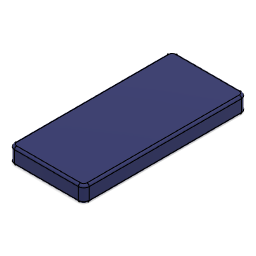
本体 v55 (Autodesk Fusion 360 archive; units mm, degrees)
design "バッテリー"
Autodesk Fusion 360 part; units mm, degrees
note: some values were not read from the file. Set by a fixed rule: which face or edge a step refers to.
sketch "スケッチ1" plane through (0, 0, 0) normal (0, 1, 0) x (1, 0, 0)
  line L0 (0, 0) -> (68.5, 0)
  line L1 (68.5, 0) -> (68.5, -149.5)
  line L2 (68.5, -149.5) -> (0, -149.5)
  line L3 (0, -149.5) -> (0, 0)
  dimension "d1" = 68.5
  dimension "d2" = 149.5
  constraint horizontal L0
  constraint vertical L1
  constraint horizontal L2
  constraint vertical L3
  constraint coincident L0.start L3.end
  measures "d1" distance of L0.start L0.end
  measures "d2" distance of L0.start L2.end
extrude "押し出し1" add sketch "スケッチ1" along normal blind 15
fillet "フィレット1" radius 5 4 edges at (68.5, 7.5, 0) (68.5, 7.5, 149.5) (0, 7.5, 149.5) (0, 7.5, 0)
fillet "フィレット2" radius 2 16 edges at (67.0355, 15, 1.4645) (34.25, 15, 0) (1.4645, 15, 1.4645) (0, 15, 74.75) (1.4645, 15, 148.0355) (34.25, 15, 149.5) (67.0355, 15, 148.0355) (68.5, 15, 74.75) (67.0355, 0, 148.0355) (34.25, 0, 149.5) (1.4645, 0, 148.0355) (0, 0, 74.75) (1.4645, 0, 1.4645) (34.25, 0, 0) (67.0355, 0, 1.4645) (68.5, 0, 74.75)
sketch "スケッチ2" plane through (0, 0, 0) normal (0, 0, -1) x (-1, 0, 0)
  line L0 (-63.5, 2) -> (-5, 2)
  line L1 (-5, 2) -> (-5, 13)
  line L2 (-5, 13) -> (-63.5, 13)
  line L3 (-63.5, 13) -> (-63.5, 2)
  line L4 (-18.8, 8.9) -> (-12.7, 8.9)
  line L5 (-11.5, 7.7) -> (-11.5, 7.3)
  line L6 (-12.7, 6.1) -> (-18.8, 6.1)
  line L7 (-20, 7.3) -> (-20, 7.7)
  line L8 (-56.5, 10.2) -> (-44.7, 10.2)
  line L9 (-44.2, 9.7) -> (-44.2, 5.3)
  line L10 (-44.7, 4.8) -> (-56.5, 4.8)
  line L11 (-57, 5.3) -> (-57, 9.7)
  line L12 (-63.5, 7.5) -> (-5, 7.5) construction
  line L13 (0, 2) -> (0, 13)
  line L14 (-68.5, 13) -> (-68.5, 2)
  arc A0 (-18.8, 8.9) -> (-20, 7.7) centre (-18.8, 7.7) ccw
  arc A1 (-20, 7.3) -> (-18.8, 6.1) centre (-18.8, 7.3) ccw
  arc A2 (-12.7, 6.1) -> (-11.5, 7.3) centre (-12.7, 7.3) ccw
  arc A3 (-11.5, 7.7) -> (-12.7, 8.9) centre (-12.7, 7.7) ccw
  arc A4 (-44.2, 9.7) -> (-44.7, 10.2) centre (-44.7, 9.7) ccw
  arc A5 (-44.7, 4.8) -> (-44.2, 5.3) centre (-44.7, 5.3) ccw
  arc A6 (-57, 5.3) -> (-56.5, 4.8) centre (-56.5, 5.3) ccw
  arc A7 (-56.5, 10.2) -> (-57, 9.7) centre (-56.5, 9.7) ccw
  point P0 (-20, 8.9)
  point P1 (-11.5, 8.9)
  point P2 (-11.5, 6.1)
  point P3 (-57, 10.2)
  point P4 (-44.2, 10.2)
  point P5 (-44.2, 4.8)
  dimension "d7" = 11.5
  dimension "d8" = 11.5
  dimension "d9" = 8.5
  dimension "d10" = 2.8
  dimension "d11" = 1.2
  dimension "d12" = 12.8
  dimension "d13" = 5.4
  dimension "d14" = 0.5
  constraint horizontal L4
  constraint vertical L5
  constraint horizontal L6
  constraint vertical L7
  constraint horizontal L8
  constraint vertical L9
  constraint horizontal L10
  constraint vertical L11
  constraint midpoint L3 L12.start
  constraint midpoint L1 L12.end
  constraint symmetric L4 L6 L12
  constraint symmetric L8 L10 L12
  constraint coincident P0 L4
  constraint coincident P0 L7
  constraint tangent L4 A0
  constraint tangent L7 A0
  constraint tangent L6 A1
  constraint tangent L7 A1
  constraint equal A0 A1
  constraint coincident P2 L5
  constraint coincident P2 L6
  constraint tangent L5 A2
  constraint tangent L6 A2
  constraint equal A0 A2
  constraint coincident P1 L4
  constraint coincident P1 L5
  constraint tangent L4 A3
  constraint tangent L5 A3
  constraint equal A0 A3
  constraint coincident P4 L8
  constraint coincident P4 L9
  constraint tangent L8 A4
  constraint tangent L9 A4
  constraint coincident P5 L9
  constraint coincident P5 L10
  constraint tangent L9 A5
  constraint tangent L10 A5
  constraint equal A4 A5
  constraint tangent L10 A6
  constraint tangent L11 A6
  constraint equal A4 A6
  constraint coincident P3 L8
  constraint coincident P3 L11
  constraint tangent L8 A7
  constraint tangent L11 A7
  constraint equal A4 A7
  measures "d7" distance of L5 L13
  measures "d8" distance of L11 L14
  measures "d9" distance of P0 P1
  measures "d10" distance of P1 P2
  measures "d11" radius of A0
  measures "d12" distance of P3 P4
  measures "d13" distance of P4 P5
  measures "d14" radius of A4
extrude "押し出し2" cut sketch "スケッチ2" against normal blind 6.5 contours L4 L5 L6 L7 A0 A1 A2 A3
extrude "押し出し3" cut sketch "スケッチ2" against normal blind 12 contours L8 L9 L10 L11 A4 A5 A6 A7

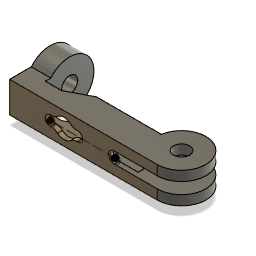
design "カメラ用マウント"
Autodesk Fusion 360 part; units mm, degrees
sketch "スケッチ1" plane through (0, 0, 0) normal (0, 1, 0) x (1, 0, 0)
  line L0 (-45.5, -7.5) -> (0, -7.5)
  circle A0 centre (0, 0) radius 2.5
  line L1 (-45.5, -7.5) -> (-45.5, 12.5)
  line L2 (-45.5, 12.5) -> (-39.5, 12.5)
  line L3 (-39.5, 12.5) -> (-39.5, -2.5)
  line L4 (-39.5, -2.5) -> (-34.5, -2.5)
  line L5 (-34.5, -2.5) -> (-27.4042, 1.1946)
  line L6 (-27.4042, 1.1946) -> (-7.4042, 1.1946)
  arc A1 (0, -7.5) -> (-7.4042, 1.1946) centre (0, 0) ccw
  line L7 (7.5, 19.5074) -> (7.5, -9) construction
  dimension "d1" = 5
  dimension "d2" = 15
  dimension "d3" = 45.5
  dimension "d4" = 20
  dimension "d5" = 6
  dimension "d6" = 5
  dimension "d7" = 8
  dimension "d8" = 20
  dimension "d9" = 5
  constraint horizontal L0
  constraint coincident A0.centre A1.centre
  constraint tangent L0 A1
  constraint perpendicular L0 L1
  constraint perpendicular L1 L2
  constraint perpendicular L2 L3
  constraint perpendicular L3 L4
  constraint parallel L4 L6
  constraint vertical L7
  constraint tangent A1 L7
  measures "d1" diameter of A0
  measures "d2" diameter of A1
  measures "d3" horizontal distance of L0.start A0.centre
  measures "d4" distance of L0 L2
  measures "d5" distance of L1.end L2.end
  measures "d6" distance of L3.end L4.end
  measures "d7" distance of L4.end L5.end
  measures "d8" distance of L5.end L6.end
  measures "d9" distance of L0 L4
extrude "押し出し1" add sketch "スケッチ1" along normal blind 9.5
sketch "スケッチ2" plane through (-45.5, 0, 0) normal (-1, 0, 0) x (0, 0, 1)
  line L0 (-12.5, 0) -> (7.5, 0)
  line L1 (7.5, 0) -> (7.5, 9.5)
  line L2 (7.5, 9.5) -> (-12.5, 9.5)
  line L3 (-12.5, 9.5) -> (-12.5, 0)
  circle A0 centre (-5, 4.75) radius 7.5
  line L4 (-12.5, 4.75) -> (7.5, 4.75) construction
  dimension "d12" = 15
  constraint tangent L3 A0
  constraint midpoint L3 L4.start
  constraint midpoint L1 L4.end
  constraint coincident A0.centre L4
  measures "d12" diameter of A0
extrude "押し出し3" cut sketch "スケッチ2" against normal up to surface (6 mm away) contours L0 L3 A0 | L2 L3 A0
extrude "押し出し2" add sketch "スケッチ2" against normal up to surface (6 mm away) contours L0 A0 | L2 A0
sketch "スケッチ3" plane through (-45.5, 0, 0) normal (-1, 0, 0) x (0, 0, 1)
  arc A0 (0.8041, 9.5) -> (0.8041, 0) centre (-5, 4.75) ccw
  line L0 (0.8041, 0) -> (7.5, 0)
  line L1 (7.5, 0) -> (7.5, 9.5)
  line L2 (7.5, 9.5) -> (0.8041, 9.5)
  circle A1 centre (-5, 4.75) radius 2.5
  dimension "d17" = 5
  constraint concentric A0 A1
  measures "d17" diameter of A1
extrude "押し出し4" cut sketch "スケッチ3" against normal up to surface (6 mm away) contours A1
sketch "スケッチ4" plane through (0, 0, 7.5) normal (0, 0, 1) x (1, 0, 0)
  line L0 (-45.5, 0) -> (0, 0)
  line L1 (0, 0) -> (0, 9.5)
  line L2 (0, 9.5) -> (-45.5, 9.5)
  line L3 (-45.5, 9.5) -> (-45.5, 0)
  line L4 (7.5, 6.5) -> (7.5, 3)
  line L5 (7.5, 3) -> (-16, 3)
  line L6 (-16, 3) -> (-13.25, 3)
  arc A0 (-13.25, 6.5) -> (-13.25, 3) centre (-13.25, 4.75) ccw
  line L7 (-13.25, 6.5) -> (7.5, 6.5)
  line L8 (0, 4.75) -> (-28.1599, 4.75) construction
  line L9 (-15, 9.5) -> (-15, 0) construction
  line L10 (7.5, 9.5) -> (-7.4042, 9.5) construction
  line L11 (7.5, 9.5) -> (7.5, 0) construction
  dimension "d20" = 3.5
  dimension "d21" = 22.5
  constraint parallel L1 L4
  constraint perpendicular L4 L5
  constraint perpendicular L4 L6
  constraint tangent L6 A0
  constraint tangent A0 L7
  constraint perpendicular L4 L7
  constraint midpoint L1 L8.start
  constraint perpendicular L1 L8
  constraint coincident L2 L9.start
  constraint coincident L0 L9.end
  constraint perpendicular L0 L9
  constraint tangent A0 L9
  constraint coincident L10.start L11.start
  constraint perpendicular L10 L11
  constraint coincident L4.start L11
  measures "d20" distance of L5 L7
  measures "d21" distance of L4 L9
extrude "押し出し5" cut sketch "スケッチ4" against normal through all contours L1 L5 A0 L7 | L1 L4 L5 L7
sketch "スケッチ5" plane through (0, 0, 7.5) normal (0, 0, 1) x (1, 0, 0)
  line L0 (0, 3) -> (-13.25, 3)
  arc A0 (-13.25, 6.5) -> (-13.25, 3) centre (-13.25, 4.75) ccw
  line L1 (-13.25, 6.5) -> (0, 6.5)
  line L2 (0, 6.5) -> (0, 9.5)
  line L3 (0, 9.5) -> (-45.5, 9.5)
  line L4 (-45.5, 9.5) -> (-45.5, 0)
  line L5 (-45.5, 0) -> (0, 0)
  line L6 (0, 0) -> (0, 3)
  line L7 (-15, 4.75) -> (-45.5, 4.75) construction
  line L8 (-23, 9.5) -> (-23, 0) construction
  line L9 (-34.5, 8.5) -> (-34.5, 0) construction
  arc A1 (-32.9093, 6.2473) -> (-32.9093, 3.2527) centre (-33, 4.75) ccw
  arc A2 (-24.5907, 3.2527) -> (-24.5907, 6.2473) centre (-24.5, 4.75) ccw
  arc A3 (-30.739, 2.5041) -> (-26.761, 2.5041) centre (-28.75, 4.75) ccw
  arc A4 (-26.761, 6.9959) -> (-30.739, 6.9959) centre (-28.75, 4.75) ccw
  arc A5 (-32.9093, 6.2473) -> (-30.739, 6.9959) centre (-32.7279, 9.2418) ccw
  arc A6 (-30.739, 2.5041) -> (-32.9093, 3.2527) centre (-32.7279, 0.2582) ccw
  arc A7 (-26.761, 6.9959) -> (-24.5907, 6.2473) centre (-24.7721, 9.2418) ccw
  arc A8 (-24.5907, 3.2527) -> (-26.761, 2.5041) centre (-24.7721, 0.2582) ccw
  dimension "d23" = 3
  dimension "d24" = 6
  dimension "d25" = 3
  dimension "d26" = 8
  dimension "d27" = 11.5
  dimension "d28" = 5.75
  dimension "d29" = 3
  constraint midpoint A0 L7.start
  constraint midpoint L4 L7.end
  constraint coincident L7 A2.centre
  constraint coincident L7 A3.centre
  constraint coincident L7 A1.centre
  constraint coincident L3 L8.start
  constraint coincident L5 L8.end
  constraint perpendicular L5 L8
  constraint tangent L8 A2
  constraint coincident L5 L9.end
  constraint perpendicular L5 L9
  constraint tangent L9 A1
  constraint concentric A3 A4
  constraint tangent A1 A5
  constraint tangent A4 A5
  constraint tangent A1 A6
  constraint tangent A3 A6
  constraint equal A5 A6
  constraint tangent A2 A7
  constraint tangent A4 A7
  constraint equal A5 A7
  constraint tangent A3 A8
  constraint tangent A2 A8
  constraint equal A5 A8
  constraint symmetric L7 A7.centre A8.centre
  measures "d23" diameter of A2
  measures "d24" diameter of A3
  measures "d25" diameter of A1
  measures "d26" distance of L7.start L8
  measures "d27" distance of L8 L9
  measures "d28" distance of A3.centre L8
  measures "d29" radius of A5
extrude "押し出し6" cut sketch "スケッチ5" against normal through all contours A1 A2 A3 A4 A5 A6 A7 A8
sketch "スケッチ6" plane through (0, 0, -1.1946) normal (0, 0, -1) x (-1, 0, 0)
  arc A0 (26.761, 2.5041) -> (27.4042, 2.0688) centre (28.75, 4.75) ccw
  arc A1 (26.761, 2.5041) -> (24.5907, 3.2527) centre (24.7721, 0.2582) ccw
  arc A2 (24.5907, 6.2473) -> (24.5907, 3.2527) centre (24.5, 4.75) ccw
  arc A3 (24.5907, 6.2473) -> (26.761, 6.9959) centre (24.7721, 9.2418) ccw
  arc A4 (27.4042, 7.4312) -> (26.761, 6.9959) centre (28.75, 4.75) ccw
  line L0 (27.4042, 7.4312) -> (27.4042, 9.5)
  line L1 (27.4042, 9.5) -> (7.4042, 9.5)
  line L2 (7.4042, 9.5) -> (7.4042, 6.5)
  line L3 (7.4042, 6.5) -> (13.25, 6.5)
  arc A5 (13.25, 3) -> (13.25, 6.5) centre (13.25, 4.75) ccw
  line L4 (13.25, 3) -> (7.4042, 3)
  line L5 (7.4042, 3) -> (7.4042, 0)
  line L6 (7.4042, 0) -> (27.4042, 0)
  line L7 (27.4042, 0) -> (27.4042, 2.0688)
  line L8 (7.4042, 8) -> (39.5, 8)
  line L9 (39.5, 8) -> (39.5, 1.5)
  line L10 (39.5, 1.5) -> (7.4042, 1.5)
  line L11 (7.4042, 1.5) -> (7.4042, 8)
  line L12 (39.5, 4.75) -> (11.4443, 4.75) construction
  line L13 (39.5, 0) -> (39.5, 9.5) construction
  point P0 (39.5, 4.75)
  dimension "d31" = 1.5
  constraint horizontal L8
  constraint vertical L9
  constraint horizontal L10
  constraint vertical L11
  constraint coincident L2 L8.start
  constraint midpoint L9 P0
  constraint perpendicular L11 L12
  constraint midpoint L13 P0
  constraint coincident P0 L12.start
  measures "d31" distance of L1 L8
extrude "押し出し7" cut sketch "スケッチ6" against normal blind 7.2 contours A0 A1 A2 A3 A4 L0 L7 L8 L9 L10 | A0 A1 A2 A3 A4 L0 L2 L3 A5 L4 L5 L7 L8 L10 L11
sketch "スケッチ7" plane through (0, 0, 7.5) normal (0, 0, 1) x (1, 0, 0)
  arc A0 (-24.5907, 3.2527) -> (-26.761, 2.5041) centre (-24.7721, 0.2582) ccw
  arc A1 (-30.739, 2.5041) -> (-26.761, 2.5041) centre (-28.75, 4.75) ccw
  arc A2 (-30.739, 2.5041) -> (-32.9093, 3.2527) centre (-32.7279, 0.2582) ccw
  arc A3 (-32.9093, 6.2473) -> (-32.9093, 3.2527) centre (-33, 4.75) ccw
  arc A4 (-32.9093, 6.2473) -> (-30.739, 6.9959) centre (-32.7279, 9.2418) ccw
  arc A5 (-26.761, 6.9959) -> (-30.739, 6.9959) centre (-28.75, 4.75) ccw
  arc A6 (-26.761, 6.9959) -> (-24.5907, 6.2473) centre (-24.7721, 9.2418) ccw
  arc A7 (-24.5907, 3.2527) -> (-24.5907, 6.2473) centre (-24.5, 4.75) ccw
  line L0 (0, 3) -> (-13.25, 3)
  arc A8 (-13.25, 6.5) -> (-13.25, 3) centre (-13.25, 4.75) ccw
  line L1 (-13.25, 6.5) -> (0, 6.5)
  line L2 (0, 6.5) -> (0, 9.5)
  line L3 (0, 9.5) -> (-45.5, 9.5)
  line L4 (-45.5, 9.5) -> (-45.5, 0)
  line L5 (-45.5, 0) -> (0, 0)
  line L6 (0, 0) -> (0, 3)
  circle A9 centre (-33, 4.75) radius 1.5 construction
  circle A10 centre (-13, 4.75) radius 1.5 construction
  line L7 (-13, 4.75) -> (-33, 4.75) construction
  dimension "d34" = 3
  dimension "d35" = 3
  dimension "d36" = 20
  constraint concentric A3 A9
  constraint coincident A10.centre L7.start
  constraint coincident A3.centre A9.centre
  constraint horizontal L7
  measures "d34" diameter of A9
  measures "d35" diameter of A10
  measures "d36" distance of A3.centre A10.centre
equation "d3 = 53 mm - 7.5 mm"
equation "d28 = ( 11.5 / 2 ) * 1 mm"

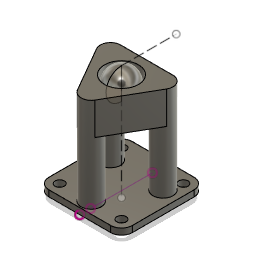
design "ボールキャスター"
Autodesk Fusion 360 part; units mm, degrees
sketch "スケッチ1" plane through (0, 0, 0) normal (0, 1, 0) x (1, 0, 0)
  line L0 (0, 0) -> (27, 0)
  line L1 (27, 0) -> (27, -27)
  line L2 (27, -27) -> (0, -27)
  line L3 (0, -27) -> (0, 0)
  dimension "d1" = 27
  dimension "d2" = 27
  constraint horizontal L0
  constraint vertical L1
  constraint horizontal L2
  constraint vertical L3
  constraint coincident L0.start L3.end
  measures "d1" distance of L0.start L2.end
  measures "d2" distance of L0.start L0.end
extrude "押し出し1" add sketch "スケッチ1" along normal blind 2
sketch "スケッチ2" plane through (0, 2, 0) normal (0, 1, 0) x (-1, 0, 0)
  line L0 (0, 27) -> (-27, 27)
  line L1 (-27, 27) -> (-27, 0)
  line L2 (-27, 0) -> (0, 0)
  line L3 (0, 0) -> (0, 27)
  circle A0 centre (-3.5, 3.5) radius 1.5
  dimension "d5" = 3
  dimension "d6" = 3.5
  dimension "d7" = 3.5
  measures "d5" diameter of A0
  measures "d6" distance of L3 A0.centre
  measures "d7" distance of L2 A0.centre
extrude "押し出し2" cut sketch "スケッチ2" against normal through all contours A0
ref_plane "作業平面1" through (13.5, 1, 15.25) normal (-1, 0, 0) x (0, 0, 1)
ref_plane "作業平面2" through (13.5, 1, 13.5) normal (0, 0, 1) x (1, 0, 0)
mirror "ミラー1" about plane through (13.5, 1, 15.25) normal (-1, 0, 0) of "押し出し2"
mirror "ミラー2" about plane through (13.5, 1, 13.5) normal (0, 0, 1) of "押し出し2", "ミラー1"
fillet "フィレット1" radius 3.5 4 edges at (27, 1, 0) (0, 1, 0) (0, 1, 27) (27, 1, 27)
sketch "スケッチ3" plane through (0, 2, 0) normal (0, 1, 0) x (-1, 0, 0)
  arc A0 (-23.5, 27) -> (-27, 23.5) centre (-23.5, 23.5) ccw
  line L0 (-27, 23.5) -> (-27, 3.5)
  arc A1 (-27, 3.5) -> (-23.5, 0) centre (-23.5, 3.5) ccw
  line L1 (-23.5, 0) -> (-3.5, 0)
  arc A2 (-3.5, 0) -> (0, 3.5) centre (-3.5, 3.5) ccw
  line L2 (0, 3.5) -> (0, 23.5)
  arc A3 (0, 23.5) -> (-3.5, 27) centre (-3.5, 23.5) ccw
  line L3 (-3.5, 27) -> (-23.5, 27)
  circle A4 centre (-23.5, 23.5) radius 1.5
  circle A5 centre (-3.5, 23.5) radius 1.5
  circle A6 centre (-23.5, 3.5) radius 1.5
  circle A7 centre (-3.5, 3.5) radius 1.5
  circle A8 centre (-22, 8.5925) radius 3.25
  circle A9 centre (-5, 8.5925) radius 3.25
  circle A10 centre (-13.5, 23.315) radius 3.25
  line L4 (-5, 8.5925) -> (-22, 8.5925) construction
  line L5 (-22, 8.5925) -> (-13.5, 23.315) construction
  line L6 (-13.5, 23.315) -> (-5, 8.5925) construction
  line L7 (0, 13.5) -> (-27, 13.5) construction
  line L8 (-13.5, 0) -> (-13.5, 27) construction
  line L9 (-5, 8.5925) -> (-17.75, 15.9537) construction
  line L10 (-22, 8.5925) -> (-9.25, 15.9537) construction
  point P0 (-13.5, 13.5)
  dimension "d12" = 6.5
  dimension "d13" = 6.5
  dimension "d14" = 6.5
  dimension "d15" = 17
  constraint coincident A9.centre L4.start
  constraint coincident A8.centre L4.end
  constraint coincident A10.centre L5.end
  constraint equal L5 L6
  constraint equal L4 L6
  constraint midpoint L2 L7.start
  constraint midpoint L0 L7.end
  constraint midpoint L1 L8.start
  constraint midpoint L3 L8.end
  constraint parallel L4 L7
  constraint coincident A10.centre L8
  constraint midpoint L5 L9.end
  constraint midpoint L6 L10.end
  constraint coincident L9 P0
  constraint coincident L10 P0
  constraint midpoint L7 P0
  measures "d12" diameter of A8
  measures "d13" diameter of A9
  measures "d14" diameter of A10
  measures "d15" distance of A8.centre A9.centre
extrude "押し出し3" add sketch "スケッチ3" along normal blind 24 contours A8 | A9 | A10
sketch "スケッチ4" plane through (0, 26, 0) normal (0, 1, 0) x (-1, 0, 0)
  circle A0 centre (-5, 8.5925) radius 3.25
  arc A1 (-5, 5.3425) -> (-2.1854, 10.2175) centre (-5, 8.5925) ccw
  line L0 (-2.1854, 10.2175) -> (-10.6854, 24.9399)
  circle A2 centre (-13.5, 23.315) radius 3.25
  arc A3 (-10.6854, 24.9399) -> (-16.3146, 24.94) centre (-13.5, 23.315) ccw
  line L1 (-5, 5.3425) -> (-22, 5.3425)
  circle A4 centre (-22, 8.5925) radius 3.25
  arc A5 (-24.8146, 10.2175) -> (-22, 5.3425) centre (-22, 8.5925) ccw
  line L2 (-24.8146, 10.2175) -> (-16.3146, 24.94)
  constraint coincident A0 A1.start
  constraint coincident A0.centre A1.centre
  constraint tangent A0 L0
  constraint tangent L0 A2
  constraint coincident A2.centre A3.centre
  constraint coincident A2 A3.end
  constraint tangent L1 A4
  constraint coincident A4 L1.end
  constraint coincident A4.centre A5.centre
  constraint tangent A4 L2
  constraint tangent A2 L2
  constraint tangent A0 L1
extrude "押し出し4" add sketch "スケッチ4" against normal blind 4
sketch "スケッチ5" plane through (13.5, 1, 15.25) normal (-1, 0, 0) x (0, 0, -1)
  line L0 (1.75, -35) -> (1.75, 1) construction
  line L1 (-11.75, -1) -> (-11.75, 1)
  line L2 (-5, -34) -> (12, -34) construction
  line L3 (11.75, 1) -> (-8.25, 1) construction
  line L4 (1.75, -34) -> (1.75, -24)
  arc A0 (1.75, -24) -> (1.75, -34) centre (1.75, -29) ccw
  dimension "d20" = 13.5
  dimension "d21" = 35
  dimension "d22" = 10
  constraint vertical L0
  constraint perpendicular L0 L2
  constraint coincident L0 L4.start
  constraint coincident L2 L4.start
  constraint perpendicular L2 L4
  constraint midpoint L4 A0.centre
  measures "d20" distance of L0 L1
  measures "d21" distance of L2 L3
  measures "d22" distance of L4.start L4.end
revolve "回転1" cut sketch "スケッチ5" angle 360 about axis through (13.5, 43.2, 13.5) along (0, -1, 0)
sketch "スケッチ6" plane through (13.5, 1, 15.25) normal (-1, 0, 0) x (0, 0, -1)
  line L0 (1.75, -34) -> (1.75, 3) construction
  line L1 (1.75, -34) -> (19.44, -34) construction
  line L2 (11.75, 1) -> (-8.25, 1)
  line L3 (1.75, -34) -> (1.75, -24)
  arc A0 (1.75, -24) -> (1.75, -34) centre (1.75, -29) ccw
  point P0 (-11.75, 1)
  dimension "d24" = 13.5
  dimension "d25" = 35
  dimension "d26" = 10
  constraint vertical L0
  constraint perpendicular L0 L1
  constraint perpendicular L1 L3
  constraint midpoint L3 A0.centre
  measures "d24" distance of L0 P0
  measures "d25" distance of L1 L2
  measures "d26" distance of L0.start L3.end
revolve "回転2" add sketch "スケッチ6" angle 360 about axis through (13.5, 43.2, 13.5) along (0, -1, 0)
sketch "スケッチ7" plane through (0, 26, 0) normal (0, 1, 0) x (-1, 0, 0)
  circle A0 centre (-13.5, 13.5) radius 3
  arc A1 (-5, 5.3425) -> (-2.1854, 10.2175) centre (-5, 8.5925) ccw
  line L0 (-2.1854, 10.2175) -> (-10.6854, 24.9399)
  arc A2 (-10.6854, 24.9399) -> (-16.3146, 24.94) centre (-13.5, 23.315) ccw
  line L1 (-16.3146, 24.94) -> (-24.8146, 10.2175)
  arc A3 (-24.8146, 10.2175) -> (-22, 5.3425) centre (-22, 8.5925) ccw
  line L2 (-22, 5.3425) -> (-5, 5.3425)
  circle A4 centre (-13.5, 13.5) radius 5.5
  arc A5 (-5, 5.3425) -> (-2.1854, 10.2175) centre (-5, 8.5925) ccw
  line L3 (-5, 5.3425) -> (-22, 5.3425)
  arc A6 (-24.8146, 10.2175) -> (-22, 5.3425) centre (-22, 8.5925) ccw
  line L4 (-24.8146, 10.2175) -> (-16.3146, 24.94)
  arc A7 (-10.6854, 24.9399) -> (-16.3146, 24.94) centre (-13.5, 23.315) ccw
  line L5 (-2.1854, 10.2175) -> (-10.6854, 24.9399)
  dimension "d28" = 11
  constraint concentric A0 A4
  measures "d28" diameter of A4
extrude "押し出し5" add sketch "スケッチ7" along normal blind 6.5 contours A1 L0 A2 L1 A3 L2 A5 L3 A6 L4 A7 L5
ref_plane "作業平面3" through (13.5, 35, 13.5) normal (0, -1, 0) x (-1, 0, 0)
equation "d20 = ( 27 / 2 ) * 1 mm"
equation "d24 = ( 27 / 2 ) * 1 mm"

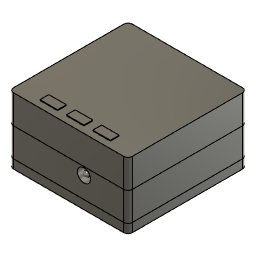
design "M5Stack"
Autodesk Fusion 360 part; units mm, degrees
sketch "スケッチ1" plane through (0, 0, 0) normal (0, 1, 0) x (1, 0, 0)
  line L0 (0, 0) -> (54, 0)
  line L1 (54, 0) -> (54, -54)
  line L2 (54, -54) -> (0, -54)
  line L3 (0, -54) -> (0, 0)
  dimension "d1" = 54
  dimension "d2" = 54
  constraint horizontal L0
  constraint vertical L1
  constraint horizontal L2
  constraint vertical L3
  constraint coincident L0.start L3.end
  measures "d1" distance of L0.start L2.end
  measures "d2" distance of L0.start L0.end
extrude "押し出し1" add sketch "スケッチ1" along normal blind 4 makes body 1
fillet "フィレット1" radius 2 4 edges at (54, 2, 54) (0, 2, 54) (54, 2, 0) (0, 2, 0) on bodies 1
sketch "スケッチ2" plane through (0, 4, 0) normal (0, 1, 0) x (-1, 0, 0)
  arc A0 (-2, 0) -> (0, 2) centre (-2, 2) ccw
  line L0 (0, 2) -> (0, 52)
  arc A1 (0, 52) -> (-2, 54) centre (-2, 52) ccw
  line L1 (-2, 54) -> (-52, 54)
  arc A2 (-52, 54) -> (-54, 52) centre (-52, 52) ccw
  line L2 (-54, 52) -> (-54, 2)
  arc A3 (-54, 2) -> (-52, 0) centre (-52, 2) ccw
  line L3 (-52, 0) -> (-2, 0)
extrude "押し出し2" add sketch "スケッチ2" along normal blind 13 separate body makes body 2
sketch "スケッチ3" plane through (0, 17, 0) normal (0, 1, 0) x (-1, 0, 0)
  line L0 (-52, 0) -> (-2, 0)
  arc A0 (-2, 0) -> (0, 2) centre (-2, 2) ccw
  line L1 (0, 2) -> (0, 52)
  arc A1 (0, 52) -> (-2, 54) centre (-2, 52) ccw
  line L2 (-2, 54) -> (-52, 54)
  arc A2 (-52, 54) -> (-54, 52) centre (-52, 52) ccw
  line L3 (-54, 52) -> (-54, 2)
  arc A3 (-54, 2) -> (-52, 0) centre (-52, 2) ccw
extrude "押し出し3" add sketch "スケッチ3" along normal blind 13 separate body makes body 3
sketch "スケッチ4" plane through (0, 30, 0) normal (0, 1, 0) x (-1, 0, 0)
  arc A0 (-54, 2) -> (-52, 0) centre (-52, 2) ccw
  line L0 (-52, 0) -> (-2, 0)
  arc A1 (-2, 0) -> (0, 2) centre (-2, 2) ccw
  line L1 (0, 2) -> (0, 52)
  arc A2 (0, 52) -> (-2, 54) centre (-2, 52) ccw
  line L2 (-2, 54) -> (-52, 54)
  arc A3 (-52, 54) -> (-54, 52) centre (-52, 52) ccw
  line L3 (-54, 52) -> (-54, 2)
  line L4 (-11, 51) -> (-19, 51)
  line L5 (-19, 51) -> (-19, 47)
  line L6 (-19, 47) -> (-11, 47)
  line L7 (-11, 47) -> (-11, 51)
  line L8 (-35, 47) -> (-43, 47)
  line L9 (-43, 47) -> (-43, 51)
  line L10 (-43, 51) -> (-35, 51)
  line L11 (-35, 51) -> (-35, 47)
  line L12 (-23, 47) -> (-31, 47)
  line L13 (-31, 47) -> (-31, 51)
  line L14 (-31, 51) -> (-23, 51)
  line L15 (-23, 51) -> (-23, 47)
  dimension "d10" = 8
  dimension "d11" = 4
  dimension "d12" = 11
  dimension "d13" = 3
  dimension "d14" = 11
  dimension "d15" = 4
  constraint horizontal L4
  constraint vertical L5
  constraint horizontal L6
  constraint vertical L7
  constraint horizontal L8
  constraint vertical L9
  constraint horizontal L10
  constraint vertical L11
  constraint horizontal L12
  constraint vertical L13
  constraint horizontal L14
  constraint vertical L15
  constraint equal L11 L15
  constraint equal L6 L12
  constraint equal L8 L12
  constraint collinear L4 L14
  constraint collinear L10 L14
  constraint equal L5 L13
  measures "d10" distance of L4.start L4.end
  measures "d11" distance of L4.start L6.end
  measures "d12" distance of L1 L7
  measures "d13" distance of L2 L4
  measures "d14" distance of L3 L9
  measures "d15" distance of L5 L15
extrude "押し出し4" add sketch "スケッチ4" along normal blind 0.3 contours L4 L5 L6 L7 | L8 L9 L10 L11 | L12 L13 L14 L15 bodies 3
fillet "フィレット2" radius 0.1 12 edges at (19, 30.15, 51) (11, 30.15, 51) (19, 30.15, 47) (11, 30.15, 47) (23, 30.15, 47) (31, 30.15, 47) (35, 30.15, 47) (23, 30.15, 51) (31, 30.15, 51) (35, 30.15, 51) (43, 30.15, 51) (43, 30.15, 47) on bodies 3
sketch "スケッチ5" plane through (0, 0, 54) normal (0, 0, 1) x (1, 0, 0)
  line L0 (2, 4) -> (52, 4)
  line L1 (52, 4) -> (52, 17)
  line L2 (52, 17) -> (2, 17)
  line L3 (2, 17) -> (2, 4)
  circle A0 centre (34, 13.5) radius 3
  line L4 (54, 4) -> (54, 17)
  dimension "d19" = 6
  dimension "d20" = 20
  dimension "d21" = 3.5
  measures "d19" diameter of A0
  measures "d20" distance of A0.centre L4
  measures "d21" distance of L2 A0.centre
extrude "押し出し5" cut sketch "スケッチ5" against normal blind 6 contours A0 bodies 2
sketch "スケッチ6" plane through (0, 0, 48) normal (0, 0, 1) x (1, 0, 0)
  circle A0 centre (34, 13.5) radius 3
  circle A1 centre (34, 13.5) radius 1.25
  dimension "d24" = 2.5
  constraint concentric A0 A1
  measures "d24" diameter of A1
extrude "押し出し6" add sketch "スケッチ6" along normal blind 6 contours A1 bodies 2
fillet "フィレット3" radius 1.25 1 edges at (32.8346, 13.048, 54) on bodies 2

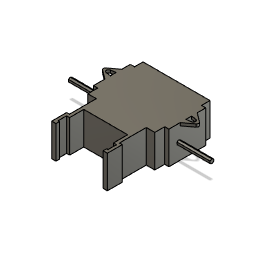
design "モーター"
Autodesk Fusion 360 part; units mm, degrees
sketch "スケッチ1" plane through (0, 0, 0) normal (0, 1, 0) x (1, 0, 0)
  line L0 (0, 0) -> (23.65, 0)
  line L1 (23.65, 0) -> (23.65, -6)
  line L2 (23.65, -6) -> (26.65, -6)
  line L3 (26.65, -6) -> (26.65, -12)
  line L4 (26.65, -24) -> (26.65, -32)
  line L5 (33.65, 3) -> (33.65, -26) construction
  line L6 (26.65, -12) -> (33.05, -16.8)
  line L7 (26.65, -24) -> (33.05, -19.2)
  arc A0 (33.05, -19.2) -> (33.05, -16.8) centre (32.15, -18) ccw
  line L8 (26.65, -32) -> (23.65, -32)
  line L9 (23.65, -32) -> (23.65, -39)
  line L10 (23.65, -39) -> (17.65, -39)
  line L11 (17.65, -39) -> (17.65, -58)
  line L12 (17.65, -58) -> (19.65, -58)
  line L13 (19.65, -58) -> (19.65, -68.5)
  line L14 (19.65, -68.5) -> (16.65, -68.5)
  line L15 (16.65, -68.5) -> (16.65, -66)
  line L16 (16.65, -66) -> (17.65, -66)
  line L17 (17.65, -66) -> (17.65, -60)
  line L18 (17.65, -60) -> (15.5083, -60)
  line L19 (15.5083, -60) -> (15.5083, -50)
  line L20 (15.5083, -50) -> (0, -50)
  line L21 (0, -50) -> (0, 0)
  dimension "d1" = 23.65
  dimension "d2" = 6
  dimension "d3" = 3
  dimension "d4" = 6
  dimension "d5" = 7
  dimension "d6" = 12
  dimension "d7" = 1.5
  dimension "d8" = 8
  dimension "d9" = 6
  dimension "d10" = 19
  dimension "d11" = 10.5
  dimension "d12" = 2
  dimension "d13" = 3
  dimension "d14" = 2
  dimension "d15" = 2.5
  dimension "d16" = 6
  dimension "d17" = 10
  dimension "d18" = 2.1417
  dimension "d19" = 7
  constraint coincident L0.start L21.end
  constraint horizontal L0
  constraint perpendicular L0 L1
  constraint perpendicular L1 L2
  constraint perpendicular L2 L3
  constraint vertical L4
  constraint collinear L3 L4
  constraint vertical L5
  constraint equal L6 L7
  constraint tangent L6 A0
  constraint tangent L7 A0
  constraint tangent L5 A0
  constraint perpendicular L4 L8
  constraint perpendicular L8 L9
  constraint perpendicular L9 L10
  constraint perpendicular L10 L11
  constraint perpendicular L9 L12
  constraint perpendicular L12 L13
  constraint equal L2 L8
  constraint perpendicular L13 L14
  constraint perpendicular L14 L15
  constraint perpendicular L15 L16
  constraint perpendicular L16 L17
  constraint perpendicular L17 L18
  constraint perpendicular L16 L19
  constraint perpendicular L19 L20
  constraint perpendicular L20 L21
  measures "d1" distance of L0.start L0.end
  measures "d2" distance of L0.end L1.end
  measures "d3" distance of L1.end L2.end
  measures "d4" distance of L2.end L3.end
  measures "d5" distance of L3 L5
  measures "d6" distance of L3.end L4.start
  measures "d7" radius of A0
  measures "d8" distance of L4.start L4.end
  measures "d9" distance of L9.end L10.end
  measures "d10" distance of L10.end L11.end
  measures "d11" distance of L12.end L13.end
  measures "d12" distance of L11.end L12.end
  measures "d13" distance of L13.end L14.end
  measures "d14" distance of L13 L17
  measures "d15" distance of L14 L16
  measures "d16" distance of L16.end L17.end
  measures "d17" distance of L18.end L19.end
  measures "d18" distance of L11 L19
  measures "d19" distance of L8.end L9.end
extrude "押し出し1" add sketch "スケッチ1" along normal blind 23 makes body 1
sketch "スケッチ2" plane through (0, 0, 0) normal (0, -1, 0) x (1, 0, 0)
  line L0 (33.05, 19.2) -> (26.65, 24)
  line L1 (26.65, 24) -> (26.65, 32)
  line L2 (26.65, 32) -> (23.65, 32)
  line L3 (23.65, 32) -> (23.65, 39)
  line L4 (23.65, 39) -> (17.65, 39)
  line L5 (17.65, 39) -> (17.65, 58)
  line L6 (17.65, 58) -> (19.65, 58)
  line L7 (19.65, 58) -> (19.65, 68.5)
  line L8 (19.65, 68.5) -> (16.65, 68.5)
  line L9 (16.65, 68.5) -> (16.65, 66)
  line L10 (16.65, 66) -> (17.65, 66)
  line L11 (17.65, 66) -> (17.65, 60)
  line L12 (17.65, 60) -> (15.5083, 60)
  line L13 (15.5083, 60) -> (15.5083, 50)
  line L14 (15.5083, 50) -> (0, 50)
  line L15 (0, 50) -> (0, 0)
  line L16 (0, 0) -> (23.65, 0)
  line L17 (23.65, 0) -> (23.65, 6)
  line L18 (23.65, 6) -> (26.65, 6)
  line L19 (26.65, 6) -> (26.65, 12)
  line L20 (26.65, 12) -> (33.05, 16.8)
  arc A0 (33.05, 16.8) -> (33.05, 19.2) centre (32.15, 18) ccw
  line L21 (26.65, 24) -> (33.05, 19.2)
  arc A1 (33.05, 16.8) -> (33.05, 19.2) centre (32.15, 18) ccw
  line L22 (26.65, 12) -> (33.05, 16.8)
  line L23 (26.65, 24) -> (26.65, 12)
  constraint coincident L0.end L1.start
  constraint coincident L19.end L20.start
extrude "押し出し2" cut sketch "スケッチ2" against normal blind 21 contours L0 L20 A0 L21 A1 L22 L23 bodies 1
sketch "スケッチ3" plane through (0, 23, 0) normal (0, 1, 0) x (-1, 0, 0)
  line L0 (-26.65, 24) -> (-33.05, 19.2)
  arc A0 (-33.05, 19.2) -> (-33.05, 16.8) centre (-32.15, 18) ccw
  line L1 (-33.05, 16.8) -> (-26.65, 12)
  line L2 (-26.65, 12) -> (-26.65, 6)
  line L3 (-26.65, 6) -> (-23.65, 6)
  line L4 (-23.65, 6) -> (-23.65, 0)
  line L5 (-23.65, 0) -> (0, 0)
  line L6 (0, 0) -> (0, 50)
  line L7 (0, 50) -> (-15.5083, 50)
  line L8 (-15.5083, 50) -> (-15.5083, 60)
  line L9 (-15.5083, 60) -> (-17.65, 60)
  line L10 (-17.65, 60) -> (-17.65, 66)
  line L11 (-17.65, 66) -> (-16.65, 66)
  line L12 (-16.65, 66) -> (-16.65, 68.5)
  line L13 (-16.65, 68.5) -> (-19.65, 68.5)
  line L14 (-19.65, 68.5) -> (-19.65, 58)
  line L15 (-19.65, 58) -> (-17.65, 58)
  line L16 (-17.65, 58) -> (-17.65, 39)
  line L17 (-17.65, 39) -> (-23.65, 39)
  line L18 (-23.65, 39) -> (-23.65, 32)
  line L19 (-23.65, 32) -> (-26.65, 32)
  line L20 (-26.65, 32) -> (-26.65, 24)
  line L21 (-32.15, 18) -> (-25, 18) construction
  line L22 (-26.65, 15.9) -> (-30.1424, 16.7262)
  arc A1 (-30.1424, 19.2738) -> (-30.1424, 16.7262) centre (-29.841, 18) ccw
  line L23 (-30.1424, 19.2738) -> (-26.65, 20.1)
  line L24 (-26.65, 20.1) -> (-26.65, 15.9)
  line L25 (-31.15, 18) -> (-31.15, 19.6) construction
  dimension "d24" = 4.2
  dimension "d25" = 4.5
  constraint coincident A0.centre L21.start
  constraint horizontal L21
  constraint tangent L22 A1
  constraint perpendicular L21 L24
  constraint collinear L2 L24
  constraint symmetric L21 L22 L23
  constraint coincident L21 A1.centre
  constraint midpoint A1 L25.start
  constraint tangent A1 L25
  constraint perpendicular L21 L25
  measures "d24" distance of L22.start L23.end
  measures "d25" distance of L24 L25
extrude "押し出し3" cut sketch "スケッチ3" against normal through all contours L22 A1 L23 L24 bodies 1
sketch "スケッチ4" plane through (26.65, 0, 0) normal (1, 0, 0) x (0, 0, -1)
  line L0 (-32, 0) -> (-6, 0)
  line L1 (-6, 0) -> (-6, 23)
  line L2 (-6, 23) -> (-12, 23)
  line L3 (-12, 23) -> (-12, 21)
  line L4 (-12, 21) -> (-15.9, 21)
  line L5 (-15.9, 21) -> (-15.9, 23)
  line L6 (-15.9, 23) -> (-20.1, 23)
  line L7 (-20.1, 23) -> (-20.1, 21)
  line L8 (-20.1, 21) -> (-24, 21)
  line L9 (-24, 21) -> (-24, 23)
  line L10 (-24, 23) -> (-32, 23)
  line L11 (-32, 23) -> (-32, 0)
  circle A0 centre (-25, 11.5) radius 1.5
  line L12 (0, 0) -> (0, 23)
  dimension "d27" = 25
  dimension "d28" = 11.5
  dimension "d29" = 3
  measures "d27" distance of A0.centre L12
  measures "d28" distance of L0 A0.centre
  measures "d29" diameter of A0
extrude "押し出し4" cut sketch "スケッチ4" along normal through all contours A0 bodies 1
sketch "スケッチ5" plane through (26.65, 0, 0) normal (1, 0, 0) x (0, 0, -1)
  circle A0 centre (-25, 11.5) radius 1.5
  line L0 (-32, 0) -> (-6, 0)
  line L1 (-6, 0) -> (-6, 23)
  line L2 (-6, 23) -> (-12, 23)
  line L3 (-12, 23) -> (-12, 21)
  line L4 (-12, 21) -> (-15.9, 21)
  line L5 (-15.9, 21) -> (-15.9, 23)
  line L6 (-15.9, 23) -> (-20.1, 23)
  line L7 (-20.1, 23) -> (-20.1, 21)
  line L8 (-20.1, 21) -> (-24, 21)
  line L9 (-24, 21) -> (-24, 23)
  line L10 (-24, 23) -> (-32, 23)
  line L11 (-32, 23) -> (-32, 0)
  line L12 (-25, 13) -> (-26.299, 12.25)
  line L13 (-26.299, 12.25) -> (-26.299, 10.75)
  line L14 (-26.299, 10.75) -> (-25, 10)
  line L15 (-25, 10) -> (-23.701, 10.75)
  line L16 (-23.701, 10.75) -> (-23.701, 12.25)
  line L17 (-23.701, 12.25) -> (-25, 13)
  line L18 (-25, 13) -> (-25, 10) construction
  point P0 (-25, 11.5)
  constraint coincident P0 A0.centre
  constraint coincident A0 L12.start
  constraint vertical L18
extrude "押し出し5" add sketch "スケッチ5" along normal blind 23.35 separate body contours L12 L13 L14 L15 L16 L17 makes body 2
sketch "スケッチ6" plane through (0, 0, 0) normal (-1, 0, 0) x (0, 0, 1)
  circle A0 centre (25, 11.5) radius 1.5
  line L0 (0, 0) -> (50, 0)
  line L1 (50, 0) -> (50, 23)
  line L2 (50, 23) -> (0, 23)
  line L3 (0, 23) -> (0, 0)
  circle A1 centre (25, 11.5) radius 1.5
extrude "押し出し6" add sketch "スケッチ6" against normal up to surface (26.65 mm away) contours A0 A1 bodies 1 2
mirror "ミラー1" about plane through (0, 0, 50) normal (-1, 0, 0) of bodies 1 makes body 3
combine "結合1" operation add target body 3 tool bodies 1
sketch "スケッチ7" plane through (0, 23, 0) normal (0, 1, 0) x (-1, 0, 0)
  line L0 (-30.1424, 19.2738) -> (-26.65, 20.1)
  line L1 (-26.65, 20.1) -> (-26.65, 15.9)
  line L2 (-26.65, 15.9) -> (-30.1424, 16.7262)
  arc A0 (-30.1424, 19.2738) -> (-30.1424, 16.7262) centre (-29.841, 18) ccw
  line L3 (26.65, 20.1) -> (30.1424, 19.2738)
  arc A1 (30.1424, 16.7262) -> (30.1424, 19.2738) centre (29.841, 18) ccw
  line L4 (30.1424, 16.7262) -> (26.65, 15.9)
  line L5 (26.65, 15.9) -> (26.65, 20.1)
  line L6 (33.05, 19.2) -> (26.65, 24)
  line L7 (26.65, 24) -> (26.65, 32)
  line L8 (26.65, 32) -> (23.65, 32)
  line L9 (23.65, 32) -> (23.65, 39)
  line L10 (23.65, 39) -> (17.65, 39)
  line L11 (17.65, 39) -> (17.65, 58)
  line L12 (17.65, 58) -> (19.65, 58)
  line L13 (19.65, 58) -> (19.65, 68.5)
  line L14 (19.65, 68.5) -> (16.65, 68.5)
  line L15 (16.65, 68.5) -> (16.65, 66)
  line L16 (16.65, 66) -> (17.65, 66)
  line L17 (17.65, 66) -> (17.65, 60)
  line L18 (17.65, 60) -> (15.5083, 60)
  line L19 (15.5083, 60) -> (15.5083, 50)
  line L20 (15.5083, 50) -> (-15.5083, 50)
  line L21 (-15.5083, 50) -> (-15.5083, 60)
  line L22 (-15.5083, 60) -> (-17.65, 60)
  line L23 (-17.65, 60) -> (-17.65, 66)
  line L24 (-17.65, 66) -> (-16.65, 66)
  line L25 (-16.65, 66) -> (-16.65, 68.5)
  line L26 (-16.65, 68.5) -> (-19.65, 68.5)
  line L27 (-19.65, 68.5) -> (-19.65, 58)
  line L28 (-19.65, 58) -> (-17.65, 58)
  line L29 (-17.65, 58) -> (-17.65, 39)
  line L30 (-17.65, 39) -> (-23.65, 39)
  line L31 (-23.65, 39) -> (-23.65, 32)
  line L32 (-23.65, 32) -> (-26.65, 32)
  line L33 (-26.65, 32) -> (-26.65, 24)
  line L34 (-26.65, 24) -> (-33.05, 19.2)
  arc A2 (-33.05, 19.2) -> (-33.05, 16.8) centre (-32.15, 18) ccw
  line L35 (-33.05, 16.8) -> (-26.65, 12)
  line L36 (-26.65, 12) -> (-26.65, 6)
  line L37 (-26.65, 6) -> (-23.65, 6)
  line L38 (-23.65, 6) -> (-23.65, 0)
  line L39 (-23.65, 0) -> (23.65, 0)
  line L40 (23.65, 0) -> (23.65, 6)
  line L41 (23.65, 6) -> (26.65, 6)
  line L42 (26.65, 6) -> (26.65, 12)
  line L43 (26.65, 12) -> (33.05, 16.8)
  arc A3 (33.05, 16.8) -> (33.05, 19.2) centre (32.15, 18) ccw
  line L44 (0, 0) -> (0, 50) construction
  line L45 (30, 18) -> (-30, 18) construction
  circle A4 centre (-30, 18) radius 1.5 construction
  circle A5 centre (-30, 18) radius 1.5
  circle A6 centre (30, 18) radius 1.5
  dimension "d36" = 60
  dimension "d37" = 3
  dimension "d38" = 3
  constraint coincident L44.start origin
  constraint midpoint L20 L44.end
  constraint horizontal L45
  constraint symmetric L44 L45.start L45.end
  constraint coincident L45.end A4.centre
  constraint concentric A4 A5
  constraint coincident L45.start A6.centre
  constraint equal A5 A6
  measures "d36" distance of L45.start L45.end
  measures "d37" diameter of A4
  measures "d38" diameter of A5
extrude "押し出し7" cut sketch "スケッチ7" against normal up to surface (2 mm away) contours L0 L2 A0 A5 | L0 L2 A0 A5 | L3 A1 L4 A6 | L3 A1 L4 A6 bodies 3
sketch "スケッチ8" plane through (0, 23, 0) normal (0, 1, 0) x (-1, 0, 0)
  line L0 (33.05, 19.2) -> (26.65, 24)
  line L1 (26.65, 24) -> (26.65, 32)
  line L2 (26.65, 32) -> (23.65, 32)
  line L3 (23.65, 32) -> (23.65, 39)
  line L4 (23.65, 39) -> (17.65, 39)
  line L5 (17.65, 39) -> (17.65, 58)
  line L6 (17.65, 58) -> (19.65, 58)
  line L7 (19.65, 58) -> (19.65, 68.5)
  line L8 (19.65, 68.5) -> (16.65, 68.5)
  line L9 (16.65, 68.5) -> (16.65, 66)
  line L10 (16.65, 66) -> (17.65, 66)
  line L11 (17.65, 66) -> (17.65, 60)
  line L12 (17.65, 60) -> (15.5083, 60)
  line L13 (15.5083, 60) -> (15.5083, 50)
  line L14 (15.5083, 50) -> (-15.5083, 50)
  line L15 (-15.5083, 50) -> (-15.5083, 60)
  line L16 (-15.5083, 60) -> (-17.65, 60)
  line L17 (-17.65, 60) -> (-17.65, 66)
  line L18 (-17.65, 66) -> (-16.65, 66)
  line L19 (-16.65, 66) -> (-16.65, 68.5)
  line L20 (-16.65, 68.5) -> (-19.65, 68.5)
  line L21 (-19.65, 68.5) -> (-19.65, 58)
  line L22 (-19.65, 58) -> (-17.65, 58)
  line L23 (-17.65, 58) -> (-17.65, 39)
  line L24 (-17.65, 39) -> (-23.65, 39)
  line L25 (-23.65, 39) -> (-23.65, 32)
  line L26 (-23.65, 32) -> (-26.65, 32)
  line L27 (-26.65, 32) -> (-26.65, 24)
  line L28 (-26.65, 24) -> (-33.05, 19.2)
  arc A0 (-33.05, 19.2) -> (-33.05, 16.8) centre (-32.15, 18) ccw
  line L29 (-33.05, 16.8) -> (-26.65, 12)
  line L30 (-26.65, 12) -> (-26.65, 6)
  line L31 (-26.65, 6) -> (-23.65, 6)
  line L32 (-23.65, 6) -> (-23.65, 0)
  line L33 (-23.65, 0) -> (23.65, 0)
  line L34 (23.65, 0) -> (23.65, 6)
  line L35 (23.65, 6) -> (26.65, 6)
  line L36 (26.65, 6) -> (26.65, 12)
  line L37 (26.65, 12) -> (33.05, 16.8)
  arc A1 (33.05, 16.8) -> (33.05, 19.2) centre (32.15, 18) ccw
  arc A2 (29.5199, 16.5789) -> (29.5199, 19.4211) centre (30, 18) ccw
  line L38 (29.5199, 16.5789) -> (26.65, 15.9)
  line L39 (26.65, 15.9) -> (26.65, 20.1)
  line L40 (26.65, 20.1) -> (29.5199, 19.4211)
  arc A3 (-29.5199, 19.4211) -> (-29.5199, 16.5789) centre (-30, 18) ccw
  line L41 (-29.5199, 19.4211) -> (-26.65, 20.1)
  line L42 (-26.65, 20.1) -> (-26.65, 15.9)
  line L43 (-26.65, 15.9) -> (-29.5199, 16.5789)
  line L44 (-26.65, 16) -> (-30.2147, 16.5154)
  line L45 (-26.65, 16) -> (-26.65, 20)
  line L46 (-26.65, 20) -> (-30.2147, 19.4846)
  arc A4 (-29.5199, 19.4211) -> (-29.5199, 16.5789) centre (-30, 18) ccw
  line L47 (-30, 18) -> (-36, 18) construction
  dimension "d41" = 4
  constraint vertical L45
  constraint collinear L42 L45
  constraint coincident A3 L46.end
  constraint tangent A3 L46
  constraint coincident L44.end A4
  constraint tangent A3 L44
  constraint coincident A3.centre A4.centre
  constraint horizontal L47
  constraint symmetric L44 L46 L47
  measures "d41" distance of L44.start L45.end
extrude "押し出し8" add sketch "スケッチ8" against normal up to surface (2 mm away) contours L41 L42 L46 | L42 L43 L44 bodies 3
extrude "押し出し9" cut sketch "スケッチ8" against normal up to surface (2 mm away) contours A3 L41 L46 A4 | A3 L43 L44 A4 bodies 3
ref_plane "作業平面1" through (0, 11.5, 19) normal (1, 0, 0) x (0, 0, -1)
mirror "ミラー2" about plane through (0, 11.5, 19) normal (1, 0, 0) of "押し出し8", "押し出し9"
equation "d1 = ( 47.3 / 2 ) * 1 mm"
